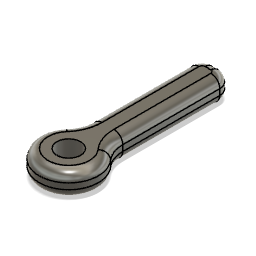
lever v8 (Autodesk Fusion 360 design; units mm, degrees)
Autodesk Fusion 360 part; units mm, degrees
sketch "Sketch1" plane through (0, 0, 0) normal (0, 1, 0) x (1, 0, 0)
  line L0 (2.5, 6.6144) -> (2.5, 23)
  line L1 (0.5, 25) -> (-0.5, 25)
  line L2 (-2.5, 23) -> (-2.5, 6.6144)
  arc A0 (-3.75, 3.3072) -> (3.75, 3.3072) centre (0, 0) ccw
  arc A1 (-3.75, 3.3072) -> (-2.5, 6.6144) centre (-7.5, 6.6144) ccw
  arc A2 (2.5, 6.6144) -> (3.75, 3.3072) centre (7.5, 6.6144) ccw
  arc A3 (-0.5, 25) -> (-2.5, 23) centre (-0.5, 23) ccw
  arc A4 (2.5, 23) -> (0.5, 25) centre (0.5, 23) ccw
  circle A5 centre (0, 0) radius 2
  dimension "d2" = 10
  dimension "d5" = 5
  dimension "d6" = 2
  constraint vertical L0
  constraint horizontal L1
  constraint vertical L2
  constraint tangent L2 A1
  constraint tangent A0 A1
  constraint tangent A0 A2
  constraint tangent L0 A2
  constraint equal A1 A2
  constraint tangent L1 A3
  constraint tangent L2 A3
  constraint tangent L0 A4
  constraint tangent L1 A4
  constraint equal A3 A4
  constraint concentric A0 A5
  measures "d2" diameter of A0
  measures "d5" radius of A1
  measures "d6" radius of A3
extrude "Estrusione9" add sketch "Sketch1" along normal blind 4
fillet "Raccordo2" radius 1.5 16 edges at (0, 4, -25) (-1.9142, 4, -24.4142) (-2.5, 4, -14.8072) (-2.8229, 4, -4.8466) (0, 4, 5) (2.8229, 4, -4.8466) (2.5, 4, -14.8072) (1.9142, 4, -24.4142) (0, 0, -25) (-1.9142, 0, -24.4142) (-2.5, 0, -14.8072) (-2.8229, 0, -4.8466) (0, 0, 5) (2.8229, 0, -4.8466) (2.5, 0, -14.8072) (1.9142, 0, -24.4142)
